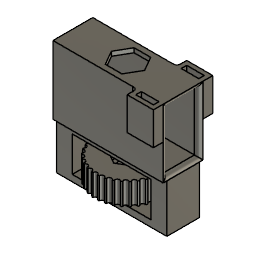
Transceiver Mounting System (Autodesk Fusion 360 design; units mm, degrees)
part number: 2025-11-02-12-33-04-707
Autodesk Fusion 360 part; units mm, degrees
sketch "Sketch1" plane through (0, 0, 0) normal (0, 0, 1) x (1, 0, 0)
  circle A0 centre (0, 0) radius 15
  dimension "d1" = 30
  constraint coincident A0.centre origin
  measures "d1" diameter of A0
extrude "Extrude1" add sketch "Sketch1" along normal blind 10 makes body 1
sketch "Sketch2" plane through (0, 0, 10) normal (0, 0, 1) x (-1, 0, 0)
  circle A0 centre (0, 0) radius 15
  circle A1 centre (0, 0) radius 3.075
  dimension "d4" = 6.15
  constraint coincident A0.centre A1.centre
  measures "d4" diameter of A1
extrude "Extrude2" cut sketch "Sketch2" against normal up to surface (10 mm away) contours A1 bodies 1
sketch "Sketch3" plane through (0, 0, 10) normal (0, 0, 1) x (-1, 0, 0)
  circle A0 centre (0, 0) radius 3.075
  circle A1 centre (0, 0) radius 15
  line L0 (0, -6.5529) -> (5.675, -3.2765)
  line L1 (5.675, -3.2765) -> (5.675, 3.2765)
  line L2 (5.675, 3.2765) -> (0, 6.5529)
  line L3 (0, 6.5529) -> (-5.675, 3.2765)
  line L4 (-5.675, 3.2765) -> (-5.675, -3.2765)
  line L5 (-5.675, -3.2765) -> (0, -6.5529)
  line L6 (0, -15) -> (0, 15) construction
  dimension "d7" = 11.35
  constraint coincident A0.centre A1.centre
  constraint coincident A1 L6.start
  constraint coincident A1 L6.end
  constraint vertical L6
  constraint coincident A0.centre L6
  constraint coincident L0.start L6
  measures "d7" distance of L2 L5
sketch "Sketch4" plane through (0, 0, 0) normal (0, 0, 1) x (1, 0, 0)
  line L0 (-23.5, 11.5) -> (23.5, 11.5)
  line L1 (23.5, 11.5) -> (23.5, -11.5)
  line L2 (23.5, -11.5) -> (-23.5, -11.5)
  line L3 (-23.5, -11.5) -> (-23.5, 11.5)
  line L4 (-23.5, 0) -> (23.5, 0) construction
  line L5 (0, 11.5) -> (0, -11.5) construction
  dimension "d8" = 23
  dimension "d9" = 47
  constraint horizontal L0
  constraint vertical L1
  constraint horizontal L2
  constraint vertical L3
  constraint midpoint L3 L4.start
  constraint midpoint L1 L4.end
  constraint coincident L4 origin
  constraint midpoint L0 L5.start
  constraint midpoint L2 L5.end
  constraint coincident origin L5
  measures "d8" distance of L0 L2
  measures "d9" distance of L1 L3
extrude "Extrude4" cut sketch "Sketch3" against normal blind 4.15 contours L0 L1 L2 L3 L4 L5 bodies 1
sketch "Sketch7" plane through (0, 0, 0) normal (0, 1, 0) x (1, 0, 0)
  line L0 (18, -13) -> (-18, -13)
  line L1 (-18, -13) -> (-18, 3)
  line L2 (-18, 3) -> (18, 3)
  line L3 (18, 3) -> (18, -13)
  line L4 (23, -16) -> (-23, -16)
  line L5 (-23, -16) -> (-23, 6)
  line L6 (-23, 6) -> (23, 6)
  line L7 (23, 6) -> (23, -16)
  line L8 (-15, -10) -> (15, -10)
  line L9 (-15, 0) -> (15, 0)
  dimension "d23" = 3
  dimension "d24" = 3
  dimension "d25" = 3
  dimension "d26" = 3
  dimension "d28" = 3
  dimension "d29" = 3
  dimension "d30" = 5
  dimension "d31" = 5
  constraint horizontal L0
  constraint vertical L1
  constraint horizontal L2
  constraint vertical L3
  constraint horizontal L4
  constraint vertical L5
  constraint horizontal L6
  constraint vertical L7
  measures "d23" distance of L3 L8.end
  measures "d24" distance of L0 L8
  measures "d25" distance of L1 L9.start
  measures "d26" distance of L2 L9
  measures "d28" distance of L0 L4
  measures "d29" distance of L2 L6
  measures "d30" distance of L3 L7
  measures "d31" distance of L1 L5
extrude "Extrude5" add sketch "Sketch7" along normal mid plane 15 separate body makes body 2
sketch "Sketch9" plane through (0, 0, 10) normal (0, 0, 1) x (-1, 0, 0)
  line L0 (5.675, -3.2765) -> (0, -6.5529)
  line L1 (0, -6.5529) -> (-5.675, -3.2765)
  line L2 (-5.675, -3.2765) -> (-5.675, 3.2765)
  line L3 (-5.675, 3.2765) -> (0, 6.5529)
  line L4 (0, 6.5529) -> (5.675, 3.2765)
  line L5 (5.675, 3.2765) -> (5.675, -3.2765)
  circle A0 centre (0, 0) radius 15
  line L6 (-6.5529, 0) -> (-3.2765, -5.675)
  line L7 (-3.2765, -5.675) -> (3.2765, -5.675)
  line L8 (3.2765, -5.675) -> (6.5529, 0)
  line L9 (6.5529, 0) -> (3.2765, 5.675)
  line L10 (3.2765, 5.675) -> (-3.2765, 5.675)
  line L11 (-3.2765, 5.675) -> (-6.5529, 0)
  line L12 (-23, 7.5) -> (-23, -7.5)
  line L13 (-23, -7.5) -> (23, -7.5)
  line L14 (23, -7.5) -> (23, 7.5)
  line L15 (23, 7.5) -> (-23, 7.5)
  line L16 (23, 0) -> (-23, 0) construction
  constraint coincident A0.centre origin
  constraint midpoint L14 L16.start
  constraint midpoint L12 L16.end
  constraint coincident L6.start L16
  constraint equal L0 L7
sketch "Sketch10" plane through (0, 0, 16) normal (0, 0, 1) x (-1, 0, 0)
  line L0 (-23, 7.5) -> (-23, -7.5)
  line L1 (-23, -7.5) -> (23, -7.5)
  line L2 (23, -7.5) -> (23, 7.5)
  line L3 (23, 7.5) -> (-23, 7.5)
  line L4 (3.2765, -5.675) -> (6.5529, 0)
  line L5 (-3.2765, -5.675) -> (3.2765, -5.675)
  line L6 (-6.5529, 0) -> (-3.2765, -5.675)
  line L7 (-3.2765, 5.675) -> (-6.5529, 0)
  line L8 (3.2765, 5.675) -> (-3.2765, 5.675)
  line L9 (6.5529, 0) -> (3.2765, 5.675)
  line L10 (-3.2765, -5.675) -> (3.2187, -5.575)
  line L11 (3.2187, -5.575) -> (6.4375, 0)
  line L12 (6.4375, 0) -> (3.2187, 5.575)
  line L13 (3.2187, 5.575) -> (-3.2187, 5.575)
  line L14 (-3.2187, 5.575) -> (-6.4375, 0)
  line L15 (-6.4375, 0) -> (-3.2765, -5.675)
  constraint coincident L5.start L6.end
extrude "Extrude6" cut sketch "Sketch10" against normal up to surface (3 mm away) contours L10 L11 L12 L13 L14 L15 bodies 2
sketch "Sketch11" plane through (0, 0, -6) normal (0, 0, -1) x (1, 0, 0)
  line L0 (-23, 7.5) -> (-23, -7.5)
  line L1 (-23, -7.5) -> (23, -7.5)
  line L2 (23, -7.5) -> (23, 7.5)
  line L3 (23, 7.5) -> (-23, 7.5)
  circle A0 centre (0, 0) radius 3.075
  circle A1 centre (0, 0) radius 15
  circle A2 centre (0, 0) radius 3.075
  constraint concentric A0 A2
  constraint equal A0 A2
extrude "Extrude7" cut sketch "Sketch11" against normal up to surface (3 mm away) contours A0 A2 bodies 2
sketch "Sketch12" plane through (0, 0, 16) normal (0, 0, 1) x (-1, 0, 0)
  line L0 (-3.2187, 5.575) -> (3.2187, 5.575)
  line L1 (3.2187, 5.575) -> (6.4375, 0)
  line L2 (6.4375, 0) -> (3.2187, -5.575)
  line L3 (3.2187, -5.575) -> (-3.2765, -5.675)
  line L4 (-3.2765, -5.675) -> (-6.4375, 0)
  line L5 (-6.4375, 0) -> (-3.2187, 5.575)
  line L6 (-23, 7.5) -> (-23, -7.5)
  line L7 (-23, -7.5) -> (23, -7.5)
  line L8 (23, -7.5) -> (23, 7.5)
  line L9 (23, 7.5) -> (-23, 7.5)
  line L10 (25.25, -9.125) -> (-25.25, -9.125)
  line L11 (-25.25, -9.125) -> (-25.25, 9.125)
  line L12 (-25.25, 9.125) -> (25.25, 9.125)
  line L13 (25.25, 9.125) -> (25.25, -9.125)
  line L14 (0, -9.125) -> (0, 9.125) construction
  line L15 (25.25, 0) -> (-25.25, 0) construction
  dimension "d38" = 18.25
  dimension "d39" = 50.5
  constraint horizontal L10
  constraint vertical L11
  constraint horizontal L12
  constraint vertical L13
  constraint midpoint L10 L14.start
  constraint midpoint L12 L14.end
  constraint midpoint L13 L15.start
  constraint midpoint L11 L15.end
  constraint coincident origin L14
  constraint coincident origin L15
  measures "d38" distance of L10.start L12.end
  measures "d39" distance of L10.start L10.end
extrude "Extrude9" add sketch "Sketch12" along normal blind 31.25 contours L6 L7 L8 L9 | L10 L11 L12 L13 bodies 2
sketch "Sketch13" plane through (25.25, 0, 0) normal (1, 0, 0) x (0, 1, 0)
  line L0 (-9.125, 16) -> (9.125, 16)
  line L1 (9.125, 16) -> (9.125, 47.25)
  line L2 (9.125, 47.25) -> (-9.125, 47.25)
  line L3 (-9.125, 47.25) -> (-9.125, 16)
  line L4 (-7.125, 45.25) -> (7.125, 45.25)
  line L5 (7.125, 45.25) -> (7.125, 18)
  line L6 (7.125, 18) -> (-7.125, 18)
  line L7 (-7.125, 18) -> (-7.125, 45.25)
  line L8 (9.125, 16) -> (-9.125, 16)
  dimension "d44" = 2
  dimension "d45" = 2
  dimension "d46" = 2
  dimension "d47" = 2
  constraint horizontal L4
  constraint vertical L5
  constraint horizontal L6
  constraint vertical L7
  measures "d44" distance of L3 L7
  measures "d45" distance of L1 L5
  measures "d46" distance of L2 L4
  measures "d47" distance of L6 L8
extrude "Extrude10" cut sketch "Sketch13" against normal up to surface (50.5 mm away) contours L4 L5 L6 L7 bodies 2
sketch "Sketch14" plane through (0, 0, 47.25) normal (0, 0, 1) x (-1, 0, 0)
  line L0 (-3.2765, -5.675) -> (-6.4375, 0)
  line L1 (-6.4375, 0) -> (-3.2187, 5.575)
  line L2 (-3.2187, 5.575) -> (3.2187, 5.575)
  line L3 (3.2187, 5.575) -> (6.4375, 0)
  line L4 (6.4375, 0) -> (3.2187, -5.575)
  line L5 (3.2187, -5.575) -> (-3.2765, -5.675)
  line L6 (25.25, 9.125) -> (-25.25, 9.125)
  line L7 (-25.25, 9.125) -> (-25.25, -9.125)
  line L8 (-25.25, -9.125) -> (25.25, -9.125)
  line L9 (25.25, -9.125) -> (25.25, 9.125)
  line L10 (-25.25, -9.125) -> (-13.25, -9.125)
  line L11 (-13.25, -9.125) -> (-13.25, -13.625)
  line L12 (-13.25, -13.625) -> (-25.25, -13.625)
  line L13 (-25.25, -13.625) -> (-25.25, -9.125)
  line L14 (-25.25, 0) -> (25.25, 0) construction
  line L15 (-13.25, 9.125) -> (-13.25, 13.625)
  line L16 (-25.25, 9.125) -> (25.25, 9.125)
  line L17 (-25.25, -9.125) -> (-25.25, 9.125)
  line L18 (-13.25, 13.625) -> (-25.25, 13.625)
  line L19 (-25.25, 13.625) -> (-25.25, 9.125)
  line L20 (-25.25, 9.125) -> (-13.25, 9.125)
  line L21 (-23.25, -9.125) -> (-15.25, -9.125)
  line L22 (-15.25, -9.125) -> (-15.25, -11.625)
  line L23 (-15.25, -11.625) -> (-23.25, -11.625)
  line L24 (-23.25, -11.625) -> (-23.25, -9.125)
  line L25 (-15.25, 9.125) -> (-15.25, 11.625)
  line L26 (-23.25, 11.625) -> (-23.25, 9.125)
  line L27 (-13.25, 13.625) -> (-25.25, 13.625)
  line L28 (-23.25, 9.125) -> (-15.25, 9.125)
  line L29 (-25.25, 13.625) -> (-25.25, 9.125)
  line L30 (-15.25, 11.625) -> (-23.25, 11.625)
  line L31 (-13.25, 9.125) -> (-13.25, 13.625)
  line L32 (-25.25, 9.125) -> (-13.25, 9.125)
  point P0 (-25.25, 9.125)
  point P1 (-25.25, 9.125)
  dimension "d50" = 12
  dimension "d51" = 4.5
  dimension "d52" = 2
  dimension "d53" = 2
  dimension "d54" = 2
  constraint horizontal L10
  constraint vertical L11
  constraint horizontal L12
  constraint vertical L13
  constraint coincident L8 L7.end
  constraint coincident L7.end L8.start
  constraint midpoint L7 L14.start
  constraint midpoint L9 L14.end
  constraint symmetric P1 L14 L7.end
  constraint symmetric L7.end L14 P1
  constraint symmetric L8.end L14 L6.start
  constraint symmetric L10.end L14 L15.start
  constraint symmetric L11.end L14 L15.end
  constraint symmetric L12.end L14 L18.end
  constraint horizontal L21
  constraint vertical L22
  constraint horizontal L23
  constraint vertical L24
  constraint coincident L10 L21.start
  constraint symmetric L14 L7.end P1
  constraint symmetric L14 L21.start L26.end
  constraint symmetric L14 L21.end L25.start
  constraint symmetric L14 L22.end L25.end
  constraint symmetric L14 L23.end L26.start
  measures "d50" distance of L11.end L12.end
  measures "d51" distance of L7.end L12.end
  measures "d52" distance of L13 L24
  measures "d53" distance of L11 L22
  measures "d54" distance of L12 L23
extrude "Extrude11" add sketch "Sketch14" against normal blind 15 contours L6 L15 L16 L18 L19 L20 L25 L26 L27 L29 L30 L31 L32 | L8 L10 L11 L12 L13 L22 L23 L24 bodies 2
ref_plane "WorkPlane1" through (0, 0, 31.625) normal (0, 1, 0) x (-1, 0, 0)
fillet "Fillet1" radius 2 tangency weight 2 2 edges at (13.25, 9.125, 39.75) (13.25, -9.125, 39.75) on bodies 2
fillet "Fillet2" radius 2 3 edges at (15.25, -10.375, 32.25) (19.25, -11.625, 32.25) (23.25, -10.375, 32.25) on bodies 2
fillet "Fillet3" radius 2 3 edges at (23.25, 10.375, 32.25) (19.25, 11.625, 32.25) (15.25, 10.375, 32.25) on bodies 2
fillet "Fillet4" radius 2 4 edges at (25.25, 0, 18) (25.25, -7.125, 31.625) (25.25, 7.125, 31.625) (25.25, 0, 45.25) on bodies 2
sketch "Sketch15" plane through (-23, 0, 0) normal (-1, 0, 0) x (0, -1, 0)
  line L0 (7.5, 16) -> (-7.5, 16)
  line L1 (-7.5, 16) -> (-7.5, -6)
  line L2 (-7.5, -6) -> (7.5, -6)
  line L3 (7.5, -6) -> (7.5, 16)
  line L4 (-7.5, 16) -> (7.5, 16)
  line L5 (7.5, 16) -> (7.5, -6)
  line L6 (7.5, -6) -> (-7.5, -6)
  line L7 (-7.5, -6) -> (-7.5, 16)
  constraint horizontal L4
  constraint vertical L5
  constraint horizontal L6
  constraint vertical L7
  constraint coincident L2.end L3.start
  constraint coincident L0.end L1.start
extrude "Extrude12" add sketch "Sketch15" along normal up to surface (2.25 mm away) bodies 2
extrude "Extrude13" add 1 faces at (23, 2.5, 8.6667) along direction (1, 0, 0) up to surface (2.25 mm away) on bodies 2 bodies 2
sketch "Sketch16" plane through (0, 0, 10) normal (0, 0, 1) x (-1, 0, 0)
  line L0 (5.675, -3.2765) -> (0, -6.5529)
  line L1 (0, -6.5529) -> (-5.675, -3.2765)
  line L2 (-5.675, -3.2765) -> (-5.675, 3.2765)
  line L3 (-5.675, 3.2765) -> (0, 6.5529)
  line L4 (0, 6.5529) -> (5.675, 3.2765)
  line L5 (5.675, 3.2765) -> (5.675, -3.2765)
  circle A0 centre (0, 0) radius 15
  circle A1 centre (0, -15) radius 1
  line L6 (0, -6.5529) -> (0, -15) construction
  circle A2 centre (2.7562, -14.7446) radius 1
  circle A3 centre (5.4186, -13.9871) radius 1
  circle A4 centre (7.8965, -12.7533) radius 1
  circle A5 centre (10.1054, -11.0851) radius 1
  circle A6 centre (11.9703, -9.0395) radius 1
  circle A7 centre (13.4274, -6.6861) radius 1
  circle A8 centre (14.4274, -4.1049) radius 1
  circle A9 centre (14.936, -1.384) radius 1
  circle A10 centre (14.936, 1.384) radius 1
  circle A11 centre (14.4274, 4.1049) radius 1
  circle A12 centre (13.4274, 6.6861) radius 1
  circle A13 centre (11.9703, 9.0395) radius 1
  circle A14 centre (10.1054, 11.0851) radius 1
  circle A15 centre (7.8965, 12.7533) radius 1
  circle A16 centre (5.4186, 13.9871) radius 1
  circle A17 centre (2.7562, 14.7446) radius 1
  circle A18 centre (0, 15) radius 1
  circle A19 centre (-2.7562, 14.7446) radius 1
  circle A20 centre (-5.4186, 13.9871) radius 1
  circle A21 centre (-7.8965, 12.7533) radius 1
  circle A22 centre (-10.1054, 11.0851) radius 1
  circle A23 centre (-11.9703, 9.0395) radius 1
  circle A24 centre (-13.4274, 6.6861) radius 1
  circle A25 centre (-14.4274, 4.1049) radius 1
  circle A26 centre (-14.936, 1.384) radius 1
  circle A27 centre (-14.936, -1.384) radius 1
  circle A28 centre (-14.4274, -4.1049) radius 1
  circle A29 centre (-13.4274, -6.6861) radius 1
  circle A30 centre (-11.9703, -9.0395) radius 1
  circle A31 centre (-10.1054, -11.0851) radius 1
  circle A32 centre (-7.8965, -12.7533) radius 1
  circle A33 centre (-5.4186, -13.9871) radius 1
  circle A34 centre (-2.7562, -14.7446) radius 1
  dimension "d69" = 2
  dimension "d71" = 360
  constraint coincident A0 A1.centre
  constraint coincident L0.end L1.start
  constraint coincident A1.centre L6.end
  constraint vertical L6
  measures "d69" diameter of A1
extrude "Extrude14" cut sketch "Sketch16" against normal up to surface (10 mm away) contours A0 A10 | A0 A9 | A0 A11 | A0 A8 | A0 A12 | A0 A7 | A0 A13 | A0 A6 | A0 A14 | A0 A5 | A0 A15 | A0 A4 | A0 A16 | A0 A3 | A0 A17 | A0 A2 | A0 A18 | A0 A1 | A0 A19 | A0 A34 | A0 A20 | A0 A33 | A0 A21 | A0 A32 | A0 A22 | A0 A31 | A0 A23 | A0 A30 | A0 A24 | A0 A29 | A0 A25 | A0 A28 | A0 A26 | A0 A27 picked at (14.6003, 1.3774) picked at (14.6003, -1.3774) picked at (14.1119, 3.9898) picked at (14.1119, -3.9898) picked at (13.1385, 6.515) picked at (13.1385, -6.515) picked at (11.7177, 8.8182) picked at (11.7177, -8.8182) picked at (9.8978, 10.8212) picked at (9.8978, -10.8212) picked at (7.7409, 12.4557) picked at (7.7409, -12.4557) picked at (5.3204, 13.666) picked at (5.3204, -13.666) picked at (2.6707, 14.4199) picked at (2.6707, -14.4199) picked at (-0.0244, 14.6651) picked at (0.0244, -14.6651) picked at (-2.6716, 14.4196) picked at (-2.6716, -14.4196) picked at (-5.2825, 13.6801) picked at (-5.2825, -13.6801) picked at (-7.7132, 12.4719) picked at (-7.7132, -12.4719) picked at (-9.8936, 10.8246) picked at (-9.8936, -10.8246) picked at (-11.6899, 8.8547) picked at (-11.6899, -8.8547) picked at (-13.122, 6.5465) picked at (-13.122, -6.5465) picked at (-14.1046, 4.0124) picked at (-14.1046, -4.0124) picked at (-14.6039, 1.3346) picked at (-14.6039, -1.3346) bodies 1
sketch "Sketch17" plane through (0, 0, -6) normal (0, 0, -1) x (1, 0, 0)
  circle A0 centre (0, 0) radius 3.075
  line L0 (-25.25, -7.5) -> (25.25, -7.5)
  line L1 (25.25, -7.5) -> (25.25, 7.5)
  line L2 (25.25, 7.5) -> (-25.25, 7.5)
  line L3 (-25.25, 7.5) -> (-25.25, -7.5)
  circle A1 centre (0, 0) radius 3.825
  dimension "d74" = 0.75
  constraint coincident A0.centre A1.centre
  measures "d74" distance of A0 A1
extrude "Extrude15" cut sketch "Sketch17" against normal up to surface (11.85 mm away) contours A1 bodies 1 2
sketch "Sketch18" plane through (0, 0, 47.25) normal (0, 0, 1) x (-1, 0, 0)
  line L0 (-25.25, 13.625) -> (-25.25, 9.125)
  line L1 (-25.25, 9.125) -> (-25.25, -9.125)
  line L2 (-25.25, -9.125) -> (-25.25, -13.625)
  line L3 (-25.25, -13.625) -> (-13.25, -13.625)
  line L4 (-13.25, -13.625) -> (-13.25, -11.125)
  spline S0 degree 3 poles (-11.25, -9.125) (-11.632, -9.125) (-11.9893, -9.1516) (-12.4665, -9.2872) (-12.6165, -9.3594) (-12.8476, -9.5381) (-12.9339, -9.6392) (-13.08, -9.892) (-13.1379, -10.0536) (-13.2304, -10.5032) (-13.25, -10.7981) (-13.25, -11.125) knots 0 0 0 0 0.114615 0.114615 0.186565 0.186565 0.250288 0.250288 0.322294 0.322294 0.415616 0.415616 0.415616 0.415616
  line L5 (-11.25, -9.125) -> (25.25, -9.125)
  line L6 (25.25, -9.125) -> (25.25, 9.125)
  line L7 (25.25, 9.125) -> (-11.25, 9.125)
  spline S1 degree 3 poles (-13.25, 11.125) (-13.25, 10.743) (-13.2234, 10.3857) (-13.0878, 9.9085) (-13.0156, 9.7585) (-12.8369, 9.5274) (-12.7358, 9.4411) (-12.483, 9.295) (-12.3214, 9.2371) (-11.8718, 9.1446) (-11.5769, 9.125) (-11.25, 9.125) knots 0 0 0 0 0.114615 0.114615 0.186565 0.186565 0.250288 0.250288 0.322294 0.322294 0.415616 0.415616 0.415616 0.415616
  line L8 (-13.25, 11.125) -> (-13.25, 13.625)
  line L9 (-13.25, 13.625) -> (-25.25, 13.625)
  line L10 (-23.25, -9.125) -> (-15.25, -9.125)
  line L11 (-15.25, -9.125) -> (-15.25, -11.625)
  line L12 (-15.25, -11.625) -> (-23.25, -11.625)
  line L13 (-23.25, -11.625) -> (-23.25, -9.125)
  line L14 (-3.2765, -5.675) -> (-6.4375, 0)
  line L15 (-6.4375, 0) -> (-3.2187, 5.575)
  line L16 (-3.2187, 5.575) -> (3.2187, 5.575)
  line L17 (3.2187, 5.575) -> (6.4375, 0)
  line L18 (6.4375, 0) -> (3.2187, -5.575)
  line L19 (3.2187, -5.575) -> (-3.2765, -5.675)
  line L20 (-23.25, 9.125) -> (-23.25, 11.625)
  line L21 (-23.25, 11.625) -> (-15.25, 11.625)
  line L22 (-15.25, 11.625) -> (-15.25, 9.125)
  line L23 (-15.25, 9.125) -> (-23.25, 9.125)
  line L24 (-3.7961, 6.575) -> (-7.5922, 0)
  line L25 (-7.5922, 0) -> (-3.7961, -6.575)
  line L26 (-3.7961, -6.575) -> (3.7961, -6.575)
  line L27 (3.7961, -6.575) -> (7.5922, 0)
  line L28 (7.5922, 0) -> (3.7961, 6.575)
  line L29 (3.7961, 6.575) -> (-3.7961, 6.575)
  line L30 (-25.25, 0) -> (25.25, 0) construction
  dimension "d77" = 13.15
  constraint midpoint L1 L30.start
  constraint midpoint L6 L30.end
  constraint coincident L24.end L30
  measures "d77" distance of L26 L29
extrude "Extrude16" cut sketch "Sketch18" against normal up to surface (34.25 mm away) contours L24 L25 L26 L27 L28 L29 bodies 2
extrude "Extrude8" [suppressed]
sketch "Sketch5" plane through (0, 0, 16) normal (0, 0, 1) x (-1, 0, 0)
  line L0 (23.5, 11.5) -> (-23.5, 11.5)
  line L1 (-23.5, 11.5) -> (-23.5, -11.5)
  line L2 (-23.5, -11.5) -> (23.5, -11.5)
  line L3 (23.5, -11.5) -> (23.5, 11.5)
sketch "Sketch6" plane through (0, -11.5, 0) normal (0, -1, 0) x (1, 0, 0)
  line L0 (23.5, -7) -> (23.5, 16)
  line L1 (23.5, 16) -> (-23.5, 16)
  line L2 (-23.5, 16) -> (-23.5, -7)
  line L3 (-23.5, -7) -> (23.5, -7)
  line L4 (-18, 13) -> (18, 13)
  line L5 (18, 13) -> (18, -3)
  line L6 (18, -3) -> (-18, -3)
  line L7 (-18, -3) -> (-18, 13)
  line L8 (15, 10) -> (-15, 10)
  line L9 (15, 0) -> (-15, 0)
  line L10 (0, 10) -> (0, 0) construction
  dimension "d14" = 3
  dimension "d15" = 3
  dimension "d16" = 3
  constraint horizontal L4
  constraint vertical L5
  constraint horizontal L6
  constraint vertical L7
  constraint midpoint L8 L10.start
  constraint coincident L10.end origin
  constraint symmetric L5 L7 L10
  measures "d14" distance of L7 L8.end
  measures "d15" distance of L4 L8
  measures "d16" distance of L6 L9
equation "d38 = 14 mm + 4.25 mm"
equation "d39 = 46.25 mm + 4.25 mm"
equation "d42 = 27 mm + 4.25 mm"
